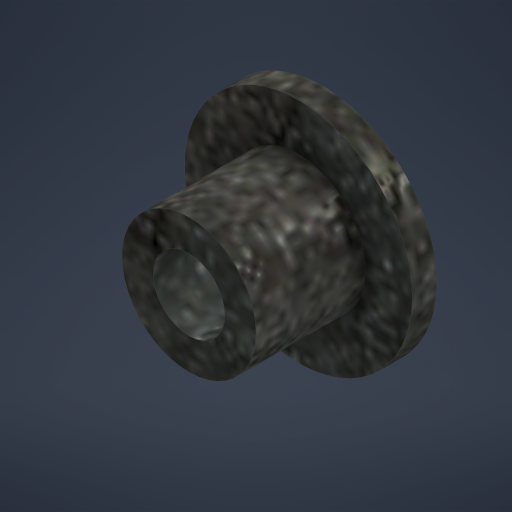
# Autodesk Inventor part: DriveSprocket
Saved by Autodesk Inventor 2024 (Build 280153000, 153)
## iProperties
Created: 2025-01-04
Part Number: DriveSprocket
Material: Steel
Document SubType Name: Modeling
Designer: Tommy Rohmann
Density: 7.85 g/cm^3
Appearance: Plate
Author: Tommy Rohmann
Autodesk Inventor part; units mm, degrees
ref_plane "YZ Plane" through (0, 0, 0) normal (1, 0, 0) x (0, 1, 0)
ref_plane "XZ Plane" through (0, 0, 0) normal (0, 1, 0) x (-1, 0, 0)
ref_plane "XY Plane" through (0, 0, 0) normal (0, 0, 1) x (1, 0, 0)
sketch "Sketch1" plane through (0, 0, 0) normal (0, 0, 1) x (1, 0, 0)
  circle A0 centre (0, 0) radius 12.7
  circle A1 centre (0, 0) radius 7.4803
  circle A2 centre (0, 0) radius 4
  dimension "d0" = 25.4
  dimension "d1" = 14.9606
  dimension "d2" = 8
  constraints: 3 centre point, 3 coincident
  measures "d0" diameter of A0
  measures "d1" diameter of A1
  measures "d2" diameter of A2
extrude "Extrusion1" add sketch "Sketch1" along normal blind 14.9479 contours A1
extrude "Extrusion2" add sketch "Sketch1" along normal blind 2.7432 contours A0
body "Solid1"
